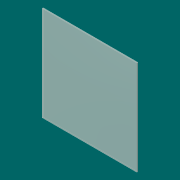
# Autodesk Inventor part: fresnelLens
Saved by Autodesk Inventor 2016 (Build 200138000, 138)
## iProperties
Created: 2015-10-13
Part Number: fresnelLens
Material: Glass
Document SubType Name: Modeling
Designer: Sawaiz
Density: 2.18 g/cm^3
Appearance: Clear
Author: Sawaiz
Autodesk Inventor part; units mm, degrees
ref_plane "YZ Plane" through (0, 0, 0) normal (1, 0, 0) x (0, 1, 0)
ref_plane "XZ Plane" through (0, 0, 0) normal (0, 1, 0) x (-1, 0, 0)
ref_plane "XY Plane" through (0, 0, 0) normal (0, 0, 1) x (1, 0, 0)
sketch "Sketch1" plane through (0, 0, 0) normal (1, 0, 0) x (0, 1, 0)
  line L0 (-85.09, -85.09) -> (85.09, -85.09)
  line L1 (85.09, -85.09) -> (85.09, 85.09)
  line L2 (85.09, 85.09) -> (-85.09, 85.09)
  line L3 (-85.09, 85.09) -> (-85.09, -85.09)
  line L4 (-85.09, -85.09) -> (85.09, 85.09) construction
  line L5 (85.09, -85.09) -> (-85.09, 85.09) construction
  point P0 (0, 0)
  dimension "d0" = 170.18
  dimension "d1" = 170.18
  constraints: 12 end point, 2 midpoint, 2 parallel, 1 horizontal, 1 perpendicular
  measures "d0" distance of L2.end L1.end
  measures "d1" distance of L1.end L0.end
extrude "Extrusion1" add sketch "Sketch1" along normal blind 1.624
ref_plane "Work Plane1" through (0, -85.09, 0) normal (0, 0, 1) x (1, 0, 0)
sketch "Sketch8" plane through (1.624, 0, 0) normal (1, 0, 0) x (0, 0, -1)
  line L0 (64.2937, -64.2937) -> (-64.2937, -64.2937)
  line L1 (-64.2937, -64.2937) -> (-64.2937, 64.2937)
  line L2 (-64.2937, 64.2937) -> (64.2937, 64.2937)
  line L3 (64.2937, 64.2937) -> (64.2937, -64.2937)
  line L4 (64.2937, -64.2937) -> (-64.2937, 64.2937) construction
  line L5 (-64.2937, -64.2937) -> (64.2937, 64.2937) construction
  point P0 (0, 0)
  dimension "d70" = 128.5875
  dimension "d71" = 128.5875
  constraints: 12 end point, 2 midpoint, 2 parallel, 1 horizontal, 1 perpendicular
  measures "d70" distance of L1.end L2.end
  measures "d71" distance of L0.end L1.end
extrude "Extrusion3" cut sketch "Sketch8" against normal through all keep common part
sketch "Sketch5" plane through (0, -85.09, 0) normal (0, 0, 1) x (1, 0, 0)
  line L0 (1.624, 0) -> (1.624, 170.18) projected
  line L1 (1.624, 85.09) -> (0, 85.09)
  arc A0 (1.624, 85.09) -> (1.524, 87.8209) centre (-35.714, 85.09) ccw
  line L2 (1.524, 87.8209) -> (1.624, 87.8209)
  line L3 (1.624, 170.18) -> (1.624, 0) projected
  arc A1 (1.624, 87.8209) -> (1.524, 88.0749) centre (-33.1682, 74.2698) ccw
  line L4 (1.524, 88.0749) -> (1.624, 88.0749)
  line L5 (-53.6482, 85.09) -> (19.5832, 85.09) projected
  line L6 (1.624, 85.09) -> (1.7573, 85.09)
  dimension "d45" = 37.338
  dimension "d47" = 0.1
  dimension "d48" = 90
  dimension "d49" = 90
  dimension "d50" = 0.254
  dimension "d51" = 0.1
  constraints: 8 end point, 4 point on circle, 3 point on line, 2 centre point, 1 equal radius, 1 horizontal, 1 midpoint, 1 tangent
  measures "d45" radius of A0
  measures "d47" distance of L2.start L2.end
  measures "d48" angle of L0 L2
  measures "d49" angle of L0 L4
  measures "d50" distance from line of L2.end L4
  measures "d51" distance of L4.start L4.end
sketch "Sketch9" plane through (0, -85.09, 0) normal (0, 0, 1) x (1, 0, 0)
  line L0 (1.624, 85.09) -> (0, 85.09)
  arc A0 (1.624, 85.09) -> (1.524, 87.9523) centre (-35.7138, 85.2184) ccw
  line L1 (1.524, 87.9523) -> (1.624, 87.9523)
  arc A1 (1.624, 87.9523) -> (1.524, 88.2063) centre (-33.1682, 74.4013) ccw
  line L2 (1.524, 88.2063) -> (1.624, 88.2063)
  line L3 (-43.1866, 85.09) -> (9.1216, 85.09)
  line L4 (1.624, 85.09) -> (1.7573, 85.09)
  line L5 (0, 20.7962) -> (0, 149.3837) projected
  line L6 (1.624, 149.3837) -> (0, 149.3837) projected
  line L7 (1.624, 149.3837) -> (1.624, 20.7962) projected
  line L8 (1.624, 20.7962) -> (0, 20.7962) projected
  line L9 (1.624, 149.3837) -> (1.624, 20.7962) projected
  point P0 (0, 85.09)
  dimension "d74" = 37.338
  dimension "d75" = 0.1
  dimension "d76" = 0.254
  dimension "d77" = 0.1
  dimension "d82" = 90
  dimension "d83" = 90
  dimension "d84" = 90
  constraints: 10 end point, 4 point on circle, 4 point on line, 3 midpoint, 2 centre point, 1 equal radius, 1 horizontal
  measures "d74" radius of A0
  measures "d75" distance of L1.start L1.end
  measures "d76" distance from line of L1.end L2
  measures "d77" distance of L2.start L2.end
  measures "d82" angle of L7 L3
  measures "d83" angle of L9 L1
  measures "d84" angle of L7 L2
equation "\"d2\" = centerThickness + fresnelThickness"
equation "\"height\" = 127"
equation "\"width\" = 127"
equation "\"fresnelThickness\" = 0.1"
equation "\"acrylicThickness\" = 6.35"
equation "\"focalLength\" = 76.2"
equation "\"ior\" = 1.49"
equation "\"fresnelAngle\" = 90deg"
equation "\"centerThickness\" = 1.524"
equation "\"fresnelChamfer\" = 6.35"
equation "\"depth\" = 146.05"
equation "\"mirrorAngle\" = 5deg"
equation "\"detectorWidth\" = 52"
equation "\"detectorHeight\" = 52"
equation "\"mirrorThickness\" = 3.175"
equation "\"fresnelEffectiveDiameter\" = 152.4"
equation "\"mirrorSuppourtWidth\" = 38.1"
equation "\"backGrooveBit\" = 4.8006"
equation "\"sensorHolderWidth\" = 88.9"
equation "\"sensorHolderHeight\" = 88.9"
equation "\"sensorHolderSensorHeight\" = 53.975"
equation "\"sensorHolderSensorWidth\" = 53.975"
equation "\"oRingWidth\" = 1.5875"
equation "\"sensorHolderORingID\" = 203.2"
equation "\"sensorHolderFlushORingID\" = 304.8"
equation "\"frontBackORingID\" = 419.1"
equation "\"mirrorGroove\" = 19.05"
equation "\"backMirrorGroove\" = 6.35"
equation "\"fresnelMirrorChamfer\" = 6.35"
equation "\"mirrorGrooveMill\" = 3.175"
equation "\"detectorOpeningHeight\" = 76.2"
equation "\"detectorOpeningWidth\" = 76.2"
equation "\"sensorHolderDepth\" = 19.05"
equation "\"frameAcrylicThickness\" = 9.525"
equation "\"internalAcrylicThicnkess\" = 6.35"
equation "\"internalAcrylicThickness\" = 6.35"
equation "\"aerogelClearence\" = 3.175"
equation "\"backplaneHoleOffsett\" = 6.35"
equation "\"backplanePCBHeight\" = 76.2"
equation "\"backplanePCBWidth\" = 76.2"
equation "\"backplanePostionOffsett\" = 12.7"
equation "\"moduleSlotClearence\" = 0.79375"
equation "\"plasticThickness\" = 6.35"
equation "\"d78\" = 0.1"
equation "\"d79\" = 76.2"
equation "\"d81\" = 1.49"
equation "\"aerogelHolderDepth\" = 37.30625"
body "Solid1"
